Autodesk Inventor part; units mm, degrees
(part 4 of 11)
  arc A1128 (24.4226, 30.9245) -> (24.4226, 30.8483) centre (24.4226, 30.8864) ccw
  arc A1129 (26.162, 30.8483) -> (26.162, 30.9245) centre (26.162, 30.8864) ccw
  line L564 (26.3694, 29.6455) -> (26.2829, 28.3315)
  arc A1130 (26.2448, 28.334) -> (26.3209, 28.329) centre (26.2829, 28.3315) ccw
  arc A1131 (26.3694, 29.6074) -> (26.3694, 29.6836) centre (26.3694, 29.6455) ccw
  line L565 (26.162, 31.0388) -> (24.8504, 31.0388)
  arc A1132 (24.8504, 31.0769) -> (24.8504, 31.0007) centre (24.8504, 31.0388) ccw
  arc A1133 (26.162, 31.0007) -> (26.162, 31.0769) centre (26.162, 31.0388) ccw
  line L566 (26.1708, 28.9489) -> (26.1308, 28.3415)
  arc A1134 (26.0928, 28.344) -> (26.1688, 28.339) centre (26.1308, 28.3415) ccw
  arc A1135 (26.1708, 28.9108) -> (26.1708, 28.987) centre (26.1708, 28.9489) ccw
  line L567 (26.162, 31.1912) -> (25.5924, 31.1912)
  arc A1136 (25.5924, 31.2293) -> (25.5924, 31.1531) centre (25.5924, 31.1912) ccw
  arc A1137 (26.162, 31.1531) -> (26.162, 31.2293) centre (26.162, 31.1912) ccw
  line L568 (5.588, 26.3398) -> (5.6423, 26.9905)
  arc A1138 (5.6803, 26.9873) -> (5.6043, 26.9937) centre (5.6423, 26.9905) ccw
  arc A1139 (5.55, 26.343) -> (5.626, 26.3366) centre (5.588, 26.3398) ccw
  line L569 (5.6423, 26.9905) -> (5.7811, 27.6286)
  arc A1140 (5.8183, 27.6205) -> (5.7439, 27.6366) centre (5.7811, 27.6286) ccw
  arc A1141 (5.6051, 26.9986) -> (5.6795, 26.9824) centre (5.6423, 26.9905) ccw
  line L570 (5.7811, 27.6286) -> (6.0019, 28.243)
  arc A1142 (6.0378, 28.2302) -> (5.9661, 28.2559) centre (6.002, 28.243) ccw
  arc A1143 (5.7452, 27.6414) -> (5.8169, 27.6157) centre (5.7811, 27.6286) ccw
  line L571 (6.0019, 28.243) -> (6.3011, 28.8234)
  arc A1144 (6.335, 28.806) -> (6.2673, 28.8409) centre (6.3011, 28.8234) ccw
  arc A1145 (5.9681, 28.2605) -> (6.0358, 28.2256) centre (6.0019, 28.243) ccw
  line L572 (6.3011, 28.8234) -> (6.6735, 29.3598)
  arc A1146 (6.7048, 29.3381) -> (6.6422, 29.3815) centre (6.6735, 29.3598) ccw
  arc A1147 (6.2698, 28.8452) -> (6.3324, 28.8017) centre (6.3011, 28.8234) ccw
  line L573 (6.6735, 29.3598) -> (7.1127, 29.843)
  arc A1148 (7.1409, 29.8174) -> (7.0845, 29.8686) centre (7.1127, 29.843) ccw
  arc A1149 (6.6453, 29.3854) -> (6.7017, 29.3342) centre (6.6735, 29.3598) ccw
  line L574 (7.1127, 29.843) -> (7.6112, 30.2647)
  arc A1150 (7.6358, 30.2356) -> (7.5866, 30.2938) centre (7.6112, 30.2647) ccw
  arc A1151 (7.0881, 29.8721) -> (7.1373, 29.8139) centre (7.1127, 29.843) ccw
  line L575 (7.6112, 30.2647) -> (8.1605, 30.6178)
  arc A1152 (8.1811, 30.5857) -> (8.1399, 30.6498) centre (8.1605, 30.6178) ccw
  arc A1153 (7.5906, 30.2968) -> (7.6318, 30.2327) centre (7.6112, 30.2647) ccw
  line L576 (8.1605, 30.6178) -> (8.7512, 30.8961)
  arc A1154 (8.7674, 30.8616) -> (8.7349, 30.9305) centre (8.7511, 30.8961) ccw
  arc A1155 (8.1443, 30.6522) -> (8.1768, 30.5833) centre (8.1605, 30.6178) ccw
  line L577 (8.7512, 30.8961) -> (9.3731, 31.0949)
  arc A1156 (9.3847, 31.0586) -> (9.3615, 31.1312) centre (9.3731, 31.0949) ccw
  arc A1157 (8.7395, 30.9324) -> (8.7627, 30.8598) centre (8.7511, 30.8961) ccw
  line L578 (9.3731, 31.0949) -> (10.0157, 31.2112)
  arc A1158 (10.0224, 31.1737) -> (10.0089, 31.2487) centre (10.0157, 31.2112) ccw
  arc A1159 (9.3663, 31.1324) -> (9.3798, 31.0574) centre (9.3731, 31.0949) ccw
  line L579 (10.0157, 31.2112) -> (10.6676, 31.2441)
  arc A1160 (10.6694, 31.206) -> (10.6658, 31.2821) centre (10.6676, 31.2441) ccw
  arc A1161 (10.0138, 31.2493) -> (10.0175, 31.1731) centre (10.0157, 31.2112) ccw
  line L580 (10.6676, 31.2441) -> (11.2768, 31.2186)
  arc A1162 (11.2731, 31.1809) -> (11.2777, 31.257) centre (11.2754, 31.2189) ccw
  arc A1163 (10.6699, 31.2821) -> (10.6653, 31.2061) centre (10.6676, 31.2441) ccw
  line L581 (11.2768, 31.2186) -> (11.8753, 31.0912)
  arc A1164 (11.8769, 31.0569) -> (11.8906, 31.1319) centre (11.8837, 31.0944) ccw
  arc A1165 (11.2822, 31.2564) -> (11.2685, 31.1815) centre (11.2754, 31.2189) ccw
  line L582 (11.8753, 31.0912) -> (12.4777, 30.9778)
  arc A1166 (12.4664, 30.9414) -> (12.489, 31.0142) centre (12.4777, 30.9778) ccw
  arc A1167 (11.8867, 31.1275) -> (11.864, 31.0548) centre (11.8753, 31.0912) ccw
  line L583 (12.4777, 30.9778) -> (12.9624, 30.6072)
  arc A1168 (12.9467, 30.5724) -> (12.978, 30.6419) centre (12.9624, 30.6072) ccw
  arc A1169 (12.4933, 31.0126) -> (12.462, 30.9431) centre (12.4777, 30.9778) ccw
  line L584 (12.9624, 30.6072) -> (14.3509, 26.7983)
  arc A1170 (14.3312, 26.7657) -> (14.3707, 26.8309) centre (14.3509, 26.7983) ccw
  arc A1171 (12.9821, 30.6398) -> (12.9427, 30.5746) centre (12.9624, 30.6072) ccw
  line L585 (14.3509, 26.7983) -> (23.3981, 15.1516)
  arc A1172 (23.4282, 15.1749) -> (23.4216, 15.1816) centre (23.3981, 15.1516) ccw
  arc A1173 (14.3744, 26.8283) -> (14.3274, 26.7683) centre (14.3509, 26.7983) ccw
  line L586 (23.3981, 15.1516) -> (19.5097, 19.7125)
  arc A1174 (16.8769, 22.7269) -> (16.8787, 22.7253) centre (16.8517, 22.6983) ccw
  arc A1175 (23.3654, 15.132) -> (23.3711, 15.1246) centre (23.3981, 15.1516) ccw
  line L587 (19.5097, 19.7125) -> (16.4438, 23.1565)
  arc A1176 (16.4139, 23.1331) -> (16.4738, 23.18) centre (16.4438, 23.1565) ccw
  arc A1177 (16.8233, 22.673) -> (16.8217, 22.6748) centre (16.8517, 22.6983) ccw
  line L588 (16.4438, 23.1565) -> (16.0942, 23.6606)
  arc A1178 (16.0616, 23.6409) -> (16.1268, 23.6803) centre (16.0942, 23.6606) ccw
  arc A1179 (16.4765, 23.1763) -> (16.4112, 23.1368) centre (16.4438, 23.1565) ccw
  line L589 (16.0942, 23.6606) -> (15.8078, 24.2031)
  arc A1180 (15.7731, 24.1874) -> (15.8426, 24.2187) centre (15.8078, 24.2031) ccw
  arc A1181 (16.1289, 23.6762) -> (16.0594, 23.6449) centre (16.0942, 23.6606) ccw
  line L590 (15.8078, 24.2031) -> (15.5889, 24.7761)
  arc A1182 (15.5525, 24.7648) -> (15.6253, 24.7875) centre (15.5889, 24.7761) ccw
  arc A1183 (15.8442, 24.2144) -> (15.7714, 24.1917) centre (15.8078, 24.2031) ccw
  line L591 (15.5889, 24.7761) -> (15.4407, 25.3714)
  arc A1184 (15.4032, 25.3645) -> (15.4781, 25.3783) centre (15.4407, 25.3714) ccw
  arc A1185 (15.6379, 27.3846) -> (15.5629, 27.3709) centre (15.6004, 27.3777) ccw
  line L592 (15.4407, 25.3714) -> (14.9039, 25.4351)
  arc A1186 (14.8659, 25.4328) -> (14.942, 25.4374) centre (14.9039, 25.4351) ccw
  arc A1187 (15.4787, 25.3737) -> (15.4026, 25.3691) centre (15.4407, 25.3714) ccw
  line L593 (14.9039, 25.4351) -> (18.8583, 22.6449)
  arc A1188 (18.8203, 22.6472) -> (18.8963, 22.6426) centre (18.8583, 22.6449) ccw
  arc A1189 (14.942, 25.4328) -> (14.8659, 25.4374) centre (14.9039, 25.4351) ccw
  line L594 (18.8583, 22.6449) -> (13.5985, 27.0666)
  arc A1190 (15.5629, 24.9531) -> (15.6379, 24.9394) centre (15.6004, 24.9463) ccw
  arc A1191 (18.8958, 22.638) -> (18.8208, 22.6517) centre (18.8583, 22.6449) ccw
  line L595 (13.5985, 27.0666) -> (5.328, 28.9324)
  arc A1192 (5.2916, 28.9437) -> (5.3643, 28.9211) centre (5.328, 28.9324) ccw
  arc A1193 (13.6349, 27.0553) -> (13.5621, 27.0779) centre (13.5985, 27.0666) ccw
  line L596 (5.328, 28.9324) -> (19.749, 27.0115)
  arc A1194 (5.9013, 28.867) -> (5.9708, 28.8358) centre (5.936, 28.8514) ccw
  arc A1195 (5.3627, 28.9167) -> (5.2932, 28.948) centre (5.328, 28.9324) ccw
  line L597 (19.749, 27.0115) -> (10.434, 29.4468)
  arc A1196 (10.4014, 29.4665) -> (10.4666, 29.4271) centre (10.434, 29.4468) ccw
  arc A1197 (19.7816, 26.9918) -> (19.7164, 27.0312) centre (19.749, 27.0115) ccw
  line L598 (10.434, 29.4468) -> (20.7175, 25.3208)
  arc A1198 (10.9892, 29.183) -> (11.0176, 29.2538) centre (11.0034, 29.2184) ccw
  arc A1199 (10.464, 29.4233) -> (10.404, 29.4703) centre (10.434, 29.4468) ccw
  line L599 (20.7175, 25.3208) -> (12.0354, 22.6782)
  arc A1200 (12.0377, 22.6402) -> (12.0332, 22.7163) centre (12.0354, 22.6782) ccw
  arc A1201 (11.0303, 29.1914) -> (10.9764, 29.2453) centre (11.0034, 29.2184) ccw
  line L600 (12.0354, 22.6782) -> (14.4431, 22.5281)
  arc A1202 (14.4196, 22.5581) -> (14.4666, 22.4982) centre (14.4431, 22.5281) ccw
  arc A1203 (12.0589, 22.6482) -> (12.0119, 22.7082) centre (12.0354, 22.6782) ccw
  line L601 (14.4431, 22.5281) -> (13.0207, 21.6798)
  arc A1204 (13.001, 21.7124) -> (13.0404, 21.6472) centre (13.0207, 21.6798) ccw
  arc A1205 (14.4628, 22.4955) -> (14.4234, 22.5608) centre (14.4431, 22.5281) ccw
  line L602 (13.0207, 21.6798) -> (12.4691, 21.4111)
  arc A1206 (12.4535, 21.4459) -> (12.4848, 21.3764) centre (12.4691, 21.4111) ccw
  arc A1207 (13.0363, 21.645) -> (13.005, 21.7145) centre (13.0207, 21.6798) ccw
  line L603 (12.4691, 21.4111) -> (11.8832, 21.2297)
  arc A1208 (11.8719, 21.2661) -> (11.8946, 21.1933) centre (11.8832, 21.2297) ccw
  arc A1209 (12.4805, 21.3748) -> (12.4578, 21.4475) centre (12.4691, 21.4111) ccw
  line L604 (11.8832, 21.2297) -> (11.28, 21.1185)
  arc A1210 (11.2731, 21.156) -> (11.2868, 21.081) centre (11.28, 21.1185) ccw
  arc A1211 (11.8906, 21.1921) -> (11.8769, 21.2671) centre (11.8837, 21.2296) ccw
  line L605 (11.28, 21.1185) -> (10.668, 21.0819)
  arc A1212 (10.6657, 21.1199) -> (10.6703, 21.0439) centre (10.668, 21.0819) ccw
  arc A1213 (11.2823, 21.0805) -> (11.2777, 21.1565) centre (11.28, 21.1185) ccw
  line L606 (10.668, 21.0819) -> (10.0106, 21.1406)
  arc A1214 (10.014, 21.1786) -> (10.0072, 21.1027) centre (10.0106, 21.1406) ccw
  arc A1215 (10.6646, 21.044) -> (10.6714, 21.1199) centre (10.668, 21.0819) ccw
  line L607 (10.0106, 21.1406) -> (9.3659, 21.2818)
  arc A1216 (9.3741, 21.319) -> (9.3578, 21.2446) centre (9.3659, 21.2818) ccw
  arc A1217 (10.0025, 21.1034) -> (10.0188, 21.1778) centre (10.0106, 21.1406) ccw
  line L608 (9.3659, 21.2818) -> (8.7436, 21.502)
  arc A1218 (8.7565, 21.5379) -> (8.7308, 21.4661) centre (8.7436, 21.502) ccw
  arc A1219 (9.3532, 21.2459) -> (9.3787, 21.3177) centre (9.3659, 21.2818) ccw
  line L609 (8.7436, 21.502) -> (8.1556, 21.8016)
  arc A1220 (8.1727, 21.8355) -> (8.1383, 21.7675) centre (8.1555, 21.8015) ccw
  arc A1221 (8.7264, 21.468) -> (8.7608, 21.536) centre (8.7436, 21.502) ccw
  line L610 (8.1556, 21.8016) -> (7.6091, 22.1716)
  arc A1222 (7.6305, 22.2032) -> (7.5877, 22.1401) centre (7.6091, 22.1716) ccw
  arc A1223 (8.1341, 21.7699) -> (8.1768, 21.833) centre (8.1555, 21.8015) ccw
  line L611 (7.6091, 22.1716) -> (7.1138, 22.6078)
  arc A1224 (7.139, 22.6364) -> (7.0887, 22.5793) centre (7.1138, 22.6078) ccw
  arc A1225 (7.5839, 22.143) -> (7.6343, 22.2002) centre (7.6091, 22.1716) ccw
  line L612 (7.1138, 22.6078) -> (6.6776, 23.1031)
  arc A1226 (6.7062, 23.1283) -> (6.649, 23.0779) centre (6.6776, 23.1031) ccw
  arc A1227 (7.0853, 22.5827) -> (7.1424, 22.633) centre (7.1138, 22.6078) ccw
  line L613 (6.6776, 23.1031) -> (6.3075, 23.6495)
  arc A1228 (6.339, 23.6708) -> (6.2759, 23.6281) centre (6.3075, 23.6495) ccw
  arc A1229 (6.6461, 23.0817) -> (6.7092, 23.1245) centre (6.6776, 23.1031) ccw
  line L614 (6.3075, 23.6495) -> (6.0093, 24.2382)
  arc A1230 (6.0432, 24.2554) -> (5.9753, 24.221) centre (6.0093, 24.2382) ccw
  arc A1231 (6.2735, 23.6323) -> (6.3415, 23.6667) centre (6.3075, 23.6495) ccw
  line L615 (6.0093, 24.2382) -> (5.7878, 24.8599)
  arc A1232 (5.8237, 24.8727) -> (5.7519, 24.8472) centre (5.7878, 24.8599) ccw
  arc A1233 (5.9734, 24.2254) -> (6.0451, 24.251) centre (6.0093, 24.2382) ccw
  line L616 (5.7878, 24.8599) -> (5.6466, 25.5046)
  arc A1234 (5.6838, 25.5128) -> (5.6094, 25.4965) centre (5.6466, 25.5046) ccw
  arc A1235 (5.7506, 24.8518) -> (5.825, 24.8681) centre (5.7878, 24.8599) ccw
  line L617 (5.6466, 25.5046) -> (5.588, 26.162)
  arc A1236 (5.6259, 26.1654) -> (5.5501, 26.1586) centre (5.588, 26.162) ccw
  arc A1237 (5.6087, 25.5012) -> (5.6846, 25.508) centre (5.6466, 25.5046) ccw
  line L618 (5.588, 26.162) -> (6.858, 26.162)
  arc A1238 (6.858, 26.1239) -> (6.858, 26.2001) centre (6.858, 26.162) ccw
  arc A1239 (5.588, 26.2001) -> (5.588, 26.1239) centre (5.588, 26.162) ccw
  line L619 (6.858, 26.162) -> (6.8774, 25.6365)
  arc A1240 (6.8393, 25.6351) -> (6.9155, 25.638) centre (6.8774, 25.6366) ccw
  arc A1241 (6.8961, 26.1634) -> (6.8199, 26.1606) centre (6.858, 26.162) ccw
  line L620 (6.8774, 25.6365) -> (6.9714, 25.1192)
  arc A1242 (6.9339, 25.1124) -> (7.0089, 25.126) centre (6.9714, 25.1192) ccw
  arc A1243 (6.9149, 25.6434) -> (6.8399, 25.6297) centre (6.8774, 25.6366) ccw
  line L621 (6.9714, 25.1192) -> (7.1381, 24.6205)
  arc A1244 (7.1019, 24.6085) -> (7.1742, 24.6326) centre (7.1381, 24.6206) ccw
  arc A1245 (7.0075, 25.1313) -> (6.9353, 25.1072) centre (6.9714, 25.1192) ccw
  line L622 (7.1381, 24.6205) -> (7.374, 24.1506)
  arc A1246 (7.34, 24.1335) -> (7.4081, 24.1677) centre (7.374, 24.1506) ccw
  arc A1247 (7.1721, 24.6376) -> (7.104, 24.6035) centre (7.1381, 24.6206) ccw
  line L623 (7.374, 24.1506) -> (7.6744, 23.7191)
  arc A1248 (7.6431, 23.6973) -> (7.7057, 23.7409) centre (7.6744, 23.7191) ccw
  arc A1249 (7.4053, 24.1724) -> (7.3427, 24.1289) centre (7.374, 24.1506) ccw
  line L624 (7.6744, 23.7191) -> (8.0332, 23.3347)
  arc A1250 (8.0053, 23.3087) -> (8.061, 23.3607) centre (8.0332, 23.3347) ccw
  arc A1251 (7.7023, 23.7451) -> (7.6465, 23.6931) centre (7.6744, 23.7191) ccw
  line L625 (8.0332, 23.3347) -> (8.443, 23.0053)
  arc A1252 (8.4191, 22.9756) -> (8.4669, 23.035) centre (8.443, 23.0053) ccw
  arc A1253 (8.057, 23.3644) -> (8.0093, 23.305) centre (8.0332, 23.3347) ccw
  line L626 (8.443, 23.0053) -> (8.8955, 22.7376)
  arc A1254 (8.8761, 22.7048) -> (8.9149, 22.7704) centre (8.8955, 22.7376) ccw
  arc A1255 (8.4624, 23.0381) -> (8.4236, 22.9725) centre (8.443, 23.0053) ccw
  line L627 (8.8955, 22.7376) -> (9.3815, 22.537)
  arc A1256 (9.367, 22.5018) -> (9.3961, 22.5722) centre (9.3815, 22.537) ccw
  arc A1257 (8.91, 22.7728) -> (8.881, 22.7024) centre (8.8955, 22.7376) ccw
  line L628 (9.3815, 22.537) -> (9.8911, 22.4076)
  arc A1258 (9.8818, 22.3706) -> (9.9005, 22.4445) centre (9.8911, 22.4076) ccw
  arc A1259 (9.3909, 22.5739) -> (9.3721, 22.5) centre (9.3815, 22.537) ccw
  line L629 (9.8911, 22.4076) -> (10.414, 22.352)
  arc A1260 (10.41, 22.3141) -> (10.418, 22.3899) centre (10.414, 22.352) ccw
  arc A1261 (9.8952, 22.4455) -> (9.8871, 22.3697) centre (9.8911, 22.4076) ccw
  line L630 (10.414, 22.352) -> (10.6681, 22.3519)
  arc A1262 (10.6681, 22.3138) -> (10.6681, 22.39) centre (10.6681, 22.3519) ccw
  arc A1263 (10.414, 22.3901) -> (10.414, 22.3139) centre (10.414, 22.352) ccw
  line L631 (10.6681, 22.3519) -> (11.2103, 22.3905)
  arc A1264 (11.213, 22.3525) -> (11.2076, 22.4285) centre (11.2103, 22.3905) ccw
  arc A1265 (10.6653, 22.3899) -> (10.6708, 22.3139) centre (10.6681, 22.3519) ccw
  line L632 (11.2103, 22.3905) -> (11.7415, 22.5058)
  arc A1266 (11.7496, 22.4686) -> (11.7334, 22.543) centre (11.7415, 22.5058) ccw
  arc A1267 (11.2022, 22.4277) -> (11.2184, 22.3532) centre (11.2103, 22.3905) ccw
  line L633 (11.7415, 22.5058) -> (12.2509, 22.6955)
  arc A1268 (12.264, 22.6606) -> (12.2374, 22.732) centre (12.2507, 22.6963) ccw
  arc A1269 (11.7282, 22.5415) -> (11.7548, 22.4701) centre (11.7415, 22.5058) ccw
  line L634 (12.2509, 22.6955) -> (12.7282, 22.9558)
  arc A1270 (12.7464, 22.9224) -> (12.7099, 22.9893) centre (12.7282, 22.9558) ccw
  arc A1271 (12.2325, 22.7297) -> (12.269, 22.6629) centre (12.2507, 22.6963) ccw
  line L635 (12.7282, 22.9558) -> (12.9175, 23.4562)
  arc A1272 (13.1859, 23.2521) -> (13.1402, 23.3131) centre (13.163, 23.2826) ccw
  arc A1273 (12.7053, 22.9863) -> (12.751, 22.9253) centre (12.7282, 22.9558) ccw
  line L636 (12.9175, 23.4562) -> (13.0355, 23.9868)
  arc A1274 (13.5743, 23.64) -> (13.5205, 23.6939) centre (13.5474, 23.667) ccw
  arc A1275 (13.1361, 23.3095) -> (13.19, 23.2557) centre (13.163, 23.2826) ccw
  line L637 (13.0355, 23.9868) -> (13.0769, 24.5288)
  arc A1276 (13.1074, 24.506) -> (13.0464, 24.5517) centre (13.0769, 24.5288) ccw
  arc A1277 (13.5169, 23.6898) -> (13.5779, 23.6441) centre (13.5474, 23.667) ccw
  line L638 (13.0769, 24.5288) -> (13.0407, 25.0712)
  arc A1278 (14.1671, 24.561) -> (14.1003, 24.5975) centre (14.1337, 24.5793) ccw
  arc A1279 (13.0435, 24.5471) -> (13.1103, 24.5106) centre (13.0769, 24.5288) ccw
  line L639 (13.0407, 25.0712) -> (12.9277, 25.6029)
  arc A1280 (12.9633, 25.5896) -> (12.892, 25.6162) centre (12.9277, 25.6029) ccw
  arc A1281 (14.098, 24.5926) -> (14.1694, 24.566) centre (14.1337, 24.5793) ccw
  line L640 (12.9277, 25.6029) -> (22.6056, 27.554)
  arc A1282 (22.6429, 27.5459) -> (22.5684, 27.5621) centre (22.6056, 27.554) ccw
  arc A1283 (12.8904, 25.611) -> (12.9649, 25.5948) centre (12.9277, 25.6029) ccw
  line L641 (22.6056, 27.554) -> (9.5434, 30.1539)
  arc A1284 (9.5814, 30.1512) -> (9.5054, 30.1566) centre (9.5434, 30.1539) ccw
  arc A1285 (22.5676, 27.5568) -> (22.6436, 27.5513) centre (22.6056, 27.554) ccw
  line L642 (9.5434, 30.1539) -> (9.9852, 30.1292)
  arc A1286 (10.0232, 30.1319) -> (9.9472, 30.1265) centre (9.9852, 30.1292) ccw
  arc A1287 (9.5054, 30.1512) -> (9.5814, 30.1566) centre (9.5434, 30.1539) ccw
  line L643 (9.9852, 30.1292) -> (10.4403, 29.8319)
  arc A1288 (10.4775, 29.84) -> (10.403, 29.8238) centre (10.4403, 29.8319) ccw
  arc A1289 (9.9479, 30.1211) -> (10.0224, 30.1373) centre (9.9852, 30.1292) ccw
  line L644 (10.4403, 29.8319) -> (10.9331, 29.6024)
  arc A1290 (14.1694, 27.758) -> (14.098, 27.7314) centre (14.1337, 27.7447) ccw
  arc A1291 (10.4046, 29.8186) -> (10.476, 29.8452) centre (10.4403, 29.8319) ccw
  line L645 (10.9331, 29.6024) -> (11.4535, 29.4454)
  arc A1292 (11.4869, 29.4637) -> (11.42, 29.4271) centre (11.4535, 29.4454) ccw
  arc A1293 (14.1003, 27.7265) -> (14.1671, 27.763) centre (14.1337, 27.7447) ccw
  line L646 (11.4535, 29.4454) -> (11.991, 29.364)
  arc A1294 (13.5779, 28.6799) -> (13.5169, 28.6342) centre (13.5474, 28.657) ccw
  arc A1295 (11.423, 29.4226) -> (11.484, 29.4682) centre (11.4535, 29.4454) ccw
  line L647 (11.991, 29.364) -> (12.5346, 29.36)
  arc A1296 (13.19, 29.0683) -> (13.1361, 29.0145) centre (13.163, 29.0414) ccw
  arc A1297 (13.5205, 28.6301) -> (13.5743, 28.684) centre (13.5474, 28.657) ccw
  line L648 (12.5346, 29.36) -> (12.7342, 29.3872)
  arc A1298 (12.7571, 29.4177) -> (12.7114, 29.3567) centre (12.7342, 29.3872) ccw
  arc A1299 (13.1402, 29.0109) -> (13.1859, 29.0719) centre (13.163, 29.0414) ccw
  line L649 (12.7342, 29.3872) -> (12.2551, 29.6441)
  arc A1300 (12.269, 29.6611) -> (12.2325, 29.5943) centre (12.2507, 29.6277) ccw
  arc A1301 (12.716, 29.3537) -> (12.7525, 29.4206) centre (12.7342, 29.3872) ccw
  line L650 (12.2551, 29.6441) -> (11.7444, 29.8301)
  arc A1302 (11.7577, 29.8658) -> (11.7311, 29.7945) centre (11.7444, 29.8301) ccw
  arc A1303 (12.2374, 29.592) -> (12.264, 29.6634) centre (12.2507, 29.6277) ccw
  line L651 (11.7444, 29.8301) -> (11.2123, 29.9416)
  arc A1304 (11.2204, 29.9789) -> (11.2042, 29.9044) centre (11.2123, 29.9416) ccw
  arc A1305 (11.7363, 29.7929) -> (11.7525, 29.8674) centre (11.7444, 29.8301) ccw
  line L652 (11.2123, 29.9416) -> (10.6698, 29.9763)
  arc A1306 (10.6726, 30.0143) -> (10.6671, 29.9383) centre (10.6698, 29.9763) ccw
  arc A1307 (11.2096, 29.9036) -> (11.2151, 29.9796) centre (11.2123, 29.9416) ccw
  line L653 (10.6698, 29.9763) -> (10.1821, 29.9523)
  arc A1308 (10.18, 29.9898) -> (10.1831, 29.9137) centre (10.1815, 29.9518) ccw
  arc A1309 (10.6714, 29.9382) -> (10.6683, 30.0144) centre (10.6698, 29.9763) ccw
  line L654 (10.1821, 29.9523) -> (9.7019, 29.8682)
  arc A1310 (9.6953, 29.9058) -> (9.7084, 29.8307) centre (9.7019, 29.8682) ccw
  arc A1311 (10.1881, 29.9142) -> (10.175, 29.9893) centre (10.1815, 29.9518) ccw
  line L655 (9.7019, 29.8682) -> (9.2372, 29.7228)
  arc A1312 (9.2258, 29.7591) -> (9.2486, 29.6864) centre (9.2372, 29.7228) ccw
  arc A1313 (9.7133, 29.8318) -> (9.6905, 29.9046) centre (9.7019, 29.8682) ccw
  line L656 (9.2372, 29.7228) -> (8.7955, 29.518)
  arc A1314 (8.7795, 29.5525) -> (8.8116, 29.4834) centre (8.7955, 29.5179) ccw
  arc A1315 (9.2533, 29.6882) -> (9.2212, 29.7573) centre (9.2372, 29.7228) ccw
  line L657 (8.7955, 29.518) -> (8.3843, 29.2572)
  arc A1316 (8.3639, 29.2894) -> (8.4047, 29.225) centre (8.3843, 29.2572) ccw
  arc A1317 (8.8159, 29.4857) -> (8.7751, 29.5501) centre (8.7955, 29.5179) ccw
  line L658 (8.3843, 29.2572) -> (8.0107, 28.945)
  arc A1318 (7.9863, 28.9742) -> (8.0352, 28.9157) centre (8.0107, 28.945) ccw
  arc A1319 (8.4088, 29.228) -> (8.3599, 29.2864) centre (8.3843, 29.2572) ccw
  line L659 (8.0107, 28.945) -> (7.6811, 28.5867)
  arc A1320 (7.653, 28.6125) -> (7.7091, 28.5609) centre (7.6811, 28.5867) ccw
  arc A1321 (8.0388, 28.9192) -> (7.9827, 28.9708) centre (8.0107, 28.945) ccw
  line L660 (7.6811, 28.5867) -> (7.401, 28.1884)
  arc A1322 (7.3698, 28.2104) -> (7.4321, 28.1665) centre (7.401, 28.1884) ccw
  arc A1323 (7.7122, 28.5648) -> (7.6499, 28.6086) centre (7.6811, 28.5867) ccw
  line L661 (7.401, 28.1884) -> (7.1753, 27.757)
  arc A1324 (7.1415, 27.7747) -> (7.209, 27.7394) centre (7.1753, 27.757) ccw
  arc A1325 (7.4347, 28.1708) -> (7.3672, 28.2061) centre (7.401, 28.1884) ccw
  line L662 (7.1753, 27.757) -> (7.6204, 27.5599)
  arc A1326 (6.972, 27.313) -> (7.0436, 27.2868) centre (7.0078, 27.2999) ccw
  arc A1327 (7.211, 27.7439) -> (7.1395, 27.7702) centre (7.1753, 27.757) ccw
  line L663 (7.6204, 27.5599) -> (6.9014, 26.8247)
  arc A1328 (6.8642, 26.8331) -> (6.9386, 26.8164) centre (6.9014, 26.8247) ccw
  arc A1329 (12.9568, 32.9698) -> (12.8825, 32.9865) centre (12.9197, 32.9781) ccw
  line L664 (6.9014, 26.8247) -> (6.858, 26.3398)
  arc A1330 (6.8201, 26.3432) -> (6.8959, 26.3364) centre (6.858, 26.3398) ccw
  arc A1331 (6.9394, 26.8213) -> (6.8635, 26.8281) centre (6.9014, 26.8247) ccw
  line L665 (6.858, 26.3398) -> (5.588, 26.3398)
  arc A1332 (5.588, 26.3779) -> (5.588, 26.3017) centre (5.588, 26.3398) ccw
  arc A1333 (6.858, 26.3017) -> (6.858, 26.3779) centre (6.858, 26.3398) ccw
  line L666 (15.4591, 25.2973) -> (14.7422, 26.1051)
  arc A1334 (14.7041, 26.1051) -> (14.7803, 26.1051) centre (14.7422, 26.1051) ccw
  arc A1335 (15.4972, 25.2973) -> (15.421, 25.2973) centre (15.4591, 25.2973) ccw
  line L667 (15.6556, 24.6016) -> (14.6713, 26.8246)
  arc A1336 (14.6332, 26.8246) -> (14.7094, 26.8246) centre (14.6713, 26.8246) ccw
  arc A1337 (15.6937, 24.6016) -> (15.6175, 24.6016) centre (15.6556, 24.6016) ccw
  line L668 (15.8368, 24.1482) -> (5.3895, 28.9242)
  arc A1338 (5.3514, 28.9242) -> (5.4276, 28.9242) centre (5.3895, 28.9242) ccw
  arc A1339 (15.8749, 24.1482) -> (15.7987, 24.1482) centre (15.8368, 24.1482) ccw
  line L669 (16.0101, 23.8198) -> (14.7162, 27.6819)
  arc A1340 (14.6781, 27.6819) -> (14.7543, 27.6819) centre (14.7162, 27.6819) ccw
  arc A1341 (16.0482, 23.8198) -> (15.972, 23.8198) centre (16.0101, 23.8198) ccw
  line L670 (16.1807, 23.5359) -> (19.6022, 27.0499)
  arc A1342 (19.5641, 27.0499) -> (19.6403, 27.0499) centre (19.6022, 27.0499) ccw
  arc A1343 (16.2188, 23.5359) -> (16.1426, 23.5359) centre (16.1807, 23.5359) ccw
  line L671 (16.3486, 23.2938) -> (14.8395, 28.295)
  arc A1344 (14.8014, 28.295) -> (14.8776, 28.295) centre (14.8395, 28.295) ccw
  arc A1345 (16.3867, 23.2938) -> (16.3105, 23.2938) centre (16.3486, 23.2938) ccw
  line L672 (16.515, 23.0767) -> (16.1422, 29.0049)
  arc A1346 (16.1041, 29.0049) -> (16.1803, 29.0049) centre (16.1422, 29.0049) ccw
  arc A1347 (16.5531, 23.0767) -> (16.4769, 23.0767) centre (16.515, 23.0767) ccw
  line L673 (16.6793, 22.8921) -> (10.7626, 29.315)
  arc A1348 (10.7245, 29.315) -> (10.8007, 29.315) centre (10.7626, 29.315) ccw
  arc A1349 (16.7174, 22.8921) -> (16.6412, 22.8921) centre (16.6793, 22.8921) ccw
  line L674 (12.0171, 28.1294) -> (9.5434, 30.1539)
  arc A1350 (9.5053, 30.1539) -> (9.5815, 30.1539) centre (9.5434, 30.1539) ccw
  arc A1351 (12.0552, 28.1294) -> (11.979, 28.1294) centre (12.0171, 28.1294) ccw
  line L675 (9.5434, 30.1539) -> (9.9028, 29.66)
  arc A1352 (9.8647, 29.66) -> (9.9409, 29.66) centre (9.9028, 29.66) ccw
  arc A1353 (9.5815, 30.1539) -> (9.5053, 30.1539) centre (9.5434, 30.1539) ccw
  line L676 (19.6426, 19.5567) -> (10.4327, 29.8369)
  arc A1354 (10.3946, 29.8369) -> (10.4708, 29.8369) centre (10.4327, 29.8369) ccw
  arc A1355 (19.6807, 19.5567) -> (19.6045, 19.5567) centre (19.6426, 19.5567) ccw
  line L677 (21.7522, 27.382) -> (20.5215, 25.2612)
  arc A1356 (20.4834, 25.2612) -> (20.5596, 25.2612) centre (20.5215, 25.2612) ccw
  arc A1357 (21.7903, 27.382) -> (21.7141, 27.382) centre (21.7522, 27.382) ccw
  line L678 (12.3669, 28.0907) -> (10.8306, 29.6501)
  arc A1358 (10.7925, 29.6501) -> (10.8687, 29.6501) centre (10.8306, 29.6501) ccw
  arc A1359 (12.405, 28.0907) -> (12.3288, 28.0907) centre (12.3669, 28.0907) ccw
  line L679 (13.0172, 25.1818) -> (14.192, 23.3346)
  arc A1360 (14.1539, 23.3346) -> (14.2301, 23.3346) centre (14.192, 23.3346) ccw
  arc A1361 (13.0553, 25.1818) -> (12.9791, 25.1818) centre (13.0172, 25.1818) ccw
  line L680 (12.58, 28.0916) -> (11.1586, 29.5344)
  arc A1362 (11.1205, 29.5344) -> (11.1967, 29.5344) centre (11.1586, 29.5344) ccw
  arc A1363 (12.6181, 28.0916) -> (12.5419, 28.0916) centre (12.58, 28.0916) ccw
  line L681 (13.0564, 24.8362) -> (14.1433, 23.1272)
  arc A1364 (14.1052, 23.1272) -> (14.1814, 23.1272) centre (14.1433, 23.1272) ccw
  arc A1365 (13.0945, 24.8362) -> (13.0183, 24.8362) centre (13.0564, 24.8362) ccw
  line L682 (23.5292, 14.9828) -> (11.4614, 29.4442)
  arc A1366 (11.4233, 29.4442) -> (11.4995, 29.4442) centre (11.4614, 29.4442) ccw
  arc A1367 (23.5673, 14.9828) -> (23.4911, 14.9828) centre (23.5292, 14.9828) ccw
  line L683 (13.0763, 24.5209) -> (12.2488, 22.6649)
  arc A1368 (12.2107, 22.6649) -> (12.2869, 22.6649) centre (12.2488, 22.6649) ccw
  arc A1369 (13.1144, 24.5209) -> (13.0382, 24.5209) centre (13.0763, 24.5209) ccw
  line L684 (23.648, 14.8299) -> (11.7128, 29.4061)
  arc A1370 (11.6747, 29.4061) -> (11.7509, 29.4061) centre (11.7128, 29.4061) ccw
  arc A1371 (23.6861, 14.8299) -> (23.6099, 14.8299) centre (23.648, 14.8299) ccw
  line L685 (13.0569, 24.2673) -> (12.442, 22.6529)
  arc A1372 (12.4039, 22.6529) -> (12.4801, 22.6529) centre (12.442, 22.6529) ccw
  arc A1373 (13.095, 24.2673) -> (13.0188, 24.2673) centre (13.0569, 24.2673) ccw
  line L686 (13.278, 28.1796) -> (11.9643, 29.3681)
  arc A1374 (11.9262, 29.3681) -> (12.0024, 29.3681) centre (11.9643, 29.3681) ccw
  arc A1375 (13.3161, 28.1796) -> (13.2399, 28.1796) centre (13.278, 28.1796) ccw
  line L687 (13.0376, 24.0137) -> (13.9419, 22.5594)
  arc A1376 (13.9038, 22.5594) -> (13.98, 22.5594) centre (13.9419, 22.5594) ccw
  arc A1377 (13.0757, 24.0137) -> (12.9995, 24.0137) centre (13.0376, 24.0137) ccw
  line L688 (14.2939, 26.9548) -> (13.2686, 25.6803)
  arc A1378 (13.2305, 25.6803) -> (13.3067, 25.6803) centre (13.2686, 25.6803) ccw
  arc A1379 (14.332, 26.9548) -> (14.2558, 26.9548) centre (14.2939, 26.9548) ccw
  line L689 (14.3098, 24.0785) -> (14.3, 22.4428)
  arc A1380 (14.2619, 22.4428) -> (14.3381, 22.4428) centre (14.3, 22.4428) ccw
  arc A1381 (14.3479, 24.0785) -> (14.2717, 24.0785) centre (14.3098, 24.0785) ccw
  line L690 (14.2329, 27.1221) -> (13.2454, 25.8946)
  arc A1382 (13.2073, 25.8946) -> (13.2835, 25.8946) centre (13.2454, 25.8946) ccw
  arc A1383 (14.271, 27.1221) -> (14.1948, 27.1221) centre (14.2329, 27.1221) ccw
  line L691 (14.1565, 23.927) -> (14.1471, 22.3516)
  arc A1384 (14.109, 22.3516) -> (14.1852, 22.3516) centre (14.1471, 22.3516) ccw
  arc A1385 (14.1946, 23.927) -> (14.1184, 23.927) centre (14.1565, 23.927) ccw
  line L692 (13.7852, 28.3501) -> (12.6046, 29.3695)
  arc A1386 (12.5665, 29.3695) -> (12.6427, 29.3695) centre (12.6046, 29.3695) ccw
  arc A1387 (13.8233, 28.3501) -> (13.7471, 28.3501) centre (13.7852, 28.3501) ccw
  line L693 (12.8925, 23.39) -> (13.6973, 22.0834)
  arc A1388 (13.6592, 22.0834) -> (13.7354, 22.0834) centre (13.6973, 22.0834) ccw
  arc A1389 (12.9306, 23.39) -> (12.8544, 23.39) centre (12.8925, 23.39) ccw
  line L694 (12.8972, 30.657) -> (12.5563, 29.2005)
  arc A1390 (12.5182, 29.2005) -> (12.5944, 29.2005) centre (12.5563, 29.2005) ccw
  arc A1391 (12.9353, 30.657) -> (12.8591, 30.657) centre (12.8972, 30.657) ccw
  line L695 (12.9015, 23.1391) -> (12.9469, 21.6439)
  arc A1392 (12.9088, 21.6439) -> (12.985, 21.6439) centre (12.9469, 21.6439) ccw
  arc A1393 (12.9396, 23.1391) -> (12.8634, 23.1391) centre (12.9015, 23.1391) ccw
  line L696 (12.7645, 30.7585) -> (12.4339, 29.3463)
  arc A1394 (12.3958, 29.3463) -> (12.472, 29.3463) centre (12.4339, 29.3463) ccw
  arc A1395 (12.8026, 30.7585) -> (12.7264, 30.7585) centre (12.7645, 30.7585) ccw
  line L697 (12.7526, 23.0204) -> (12.7967, 21.5707)
  arc A1396 (12.7586, 21.5707) -> (12.8348, 21.5707) centre (12.7967, 21.5707) ccw
  arc A1397 (12.7907, 23.0204) -> (12.7145, 23.0204) centre (12.7526, 23.0204) ccw
  line L698 (12.6444, 30.8503) -> (12.6553, 29.4295)
  arc A1398 (12.6172, 29.4295) -> (12.6934, 29.4295) centre (12.6553, 29.4295) ccw
  arc A1399 (12.6825, 30.8503) -> (12.6063, 30.8503) centre (12.6444, 30.8503) ccw
  line L699 (12.6495, 22.9129) -> (12.6464, 21.4975)
  arc A1400 (12.6083, 21.4975) -> (12.6845, 21.4975) centre (12.6464, 21.4975) ccw
  arc A1401 (12.6876, 22.9129) -> (12.6114, 22.9129) centre (12.6495, 22.9129) ccw
  line L700 (12.4915, 30.9178) -> (12.5022, 29.5116)
  arc A1402 (12.4641, 29.5116) -> (12.5403, 29.5116) centre (12.5022, 29.5116) ccw
  arc A1403 (12.5296, 30.9178) -> (12.4534, 30.9178) centre (12.4915, 30.9178) ccw
  line L701 (12.4971, 22.8298) -> (12.4962, 21.4243)
  arc A1404 (12.4581, 21.4243) -> (12.5343, 21.4243) centre (12.4962, 21.4243) ccw
  arc A1405 (12.5352, 22.8298) -> (12.459, 22.8298) centre (12.4971, 22.8298) ccw
  line L702 (12.3387, 30.9679) -> (12.3492, 29.5936)
  arc A1406 (12.3111, 29.5936) -> (12.3873, 29.5936) centre (12.3492, 29.5936) ccw
  arc A1407 (12.3768, 30.9679) -> (12.3006, 30.9679) centre (12.3387, 30.9679) ccw
  line L703 (12.3446, 22.7466) -> (12.344, 21.3723)
  arc A1408 (12.3059, 21.3723) -> (12.3821, 21.3723) centre (12.344, 21.3723) ccw
  arc A1409 (12.3827, 22.7466) -> (12.3065, 22.7466) centre (12.3446, 22.7466) ccw
  line L704 (12.1921, 31.0316) -> (12.1963, 29.6655)
  arc A1410 (12.1582, 29.6655) -> (12.2344, 29.6655) centre (12.1963, 29.6655) ccw
  arc A1411 (12.2302, 31.0316) -> (12.154, 31.0316) centre (12.1921, 31.0316) ccw
  line L705 (12.1922, 22.6736) -> (12.1916, 21.3252)
  arc A1412 (12.1535, 21.3252) -> (12.2297, 21.3252) centre (12.1916, 21.3252) ccw
  arc A1413 (12.2303, 22.6736) -> (12.1541, 22.6736) centre (12.1922, 22.6736) ccw
  line L706 (12.0334, 31.0614) -> (12.0434, 29.7212)
  arc A1414 (12.0053, 29.7212) -> (12.0815, 29.7212) centre (12.0434, 29.7212) ccw
  arc A1415 (12.0715, 31.0614) -> (11.9953, 31.0614) centre (12.0334, 31.0614) ccw
  line L707 (12.0398, 22.6169) -> (12.039, 21.2779)
  arc A1416 (12.0009, 21.2779) -> (12.0771, 21.2779) centre (12.039, 21.2779) ccw
  arc A1417 (12.0779, 22.6169) -> (12.0017, 22.6169) centre (12.0398, 22.6169) ccw
  line L708 (11.8805, 31.1069) -> (11.8906, 29.7769)
  arc A1418 (11.8525, 29.7769) -> (11.9287, 29.7769) centre (11.8906, 29.7769) ccw
  arc A1419 (11.9186, 31.1069) -> (11.8424, 31.1069) centre (11.8805, 31.1069) ccw
  line L709 (11.8874, 22.5601) -> (11.8867, 21.2301)
  arc A1420 (11.8486, 21.2301) -> (11.9248, 21.2301) centre (11.8867, 21.2301) ccw
  arc A1421 (11.9255, 22.5601) -> (11.8493, 22.5601) centre (11.8874, 22.5601) ccw
  line L710 (11.7348, 31.1217) -> (11.7348, 29.8191)
  arc A1422 (11.6967, 29.8191) -> (11.7729, 29.8191) centre (11.7348, 29.8191) ccw
  arc A1423 (11.7729, 31.1217) -> (11.6967, 31.1217) centre (11.7348, 31.1217) ccw
  line L711 (11.7348, 22.5049) -> (11.7348, 21.2023)
  arc A1424 (11.6967, 21.2023) -> (11.7729, 21.2023) centre (11.7348, 21.2023) ccw
  arc A1425 (11.7729, 22.5049) -> (11.6967, 22.5049) centre (11.7348, 22.5049) ccw
  line L712 (11.5757, 31.155) -> (11.5851, 29.8635)
  arc A1426 (11.547, 29.8635) -> (11.6232, 29.8635) centre (11.5851, 29.8635) ccw
  arc A1427 (11.6138, 31.155) -> (11.5376, 31.155) centre (11.5757, 31.155) ccw
  line L713 (11.5825, 22.4713) -> (11.582, 21.1742)
  arc A1428 (11.5439, 21.1742) -> (11.6201, 21.1742) centre (11.582, 21.1742) ccw
  arc A1429 (11.6206, 22.4713) -> (11.5444, 22.4713) centre (11.5825, 22.4713) ccw
  line L714 (11.4226, 31.1876) -> (11.4325, 29.8955)
  arc A1430 (11.3944, 29.8955) -> (11.4706, 29.8955) centre (11.4325, 29.8955) ccw
  arc A1431 (11.4607, 31.1876) -> (11.3845, 31.1876) centre (11.4226, 31.1876) ccw
  line L715 (11.4301, 22.4382) -> (11.4295, 21.1461)
  arc A1432 (11.3914, 21.1461) -> (11.4676, 21.1461) centre (11.4295, 21.1461) ccw
  arc A1433 (11.4682, 22.4382) -> (11.392, 22.4382) centre (11.4301, 22.4382) ccw
  line L716 (11.27, 31.214) -> (11.2798, 29.9275)
  arc A1434 (11.2417, 29.9275) -> (11.3179, 29.9275) centre (11.2798, 29.9275) ccw
  arc A1435 (11.3081, 31.214) -> (11.2319, 31.214) centre (11.27, 31.214) ccw
  line L717 (11.2777, 22.4051) -> (11.2771, 21.1186)
  arc A1436 (11.239, 21.1186) -> (11.3152, 21.1186) centre (11.2771, 21.1186) ccw
  arc A1437 (11.3158, 22.4051) -> (11.2396, 22.4051) centre (11.2777, 22.4051) ccw
  line L718 (11.1215, 31.2251) -> (11.1453, 29.9503)
  arc A1438 (11.1072, 29.9503) -> (11.1834, 29.9503) centre (11.1453, 29.9503) ccw
  arc A1439 (11.1596, 31.2251) -> (11.0834, 31.2251) centre (11.1215, 31.2251) ccw
  line L719 (11.1258, 22.3843) -> (11.1249, 21.1092)
  arc A1440 (11.0868, 21.1092) -> (11.163, 21.1092) centre (11.1249, 21.1092) ccw
  arc A1441 (11.1639, 22.3843) -> (11.0877, 22.3843) centre (11.1258, 22.3843) ccw
  line L720 (10.969, 31.2315) -> (10.9748, 29.9568)
  arc A1442 (10.9367, 29.9568) -> (11.0129, 29.9568) centre (10.9748, 29.9568) ccw
  arc A1443 (11.0071, 31.2315) -> (10.9309, 31.2315) centre (10.969, 31.2315) ccw
  line L721 (10.9729, 22.3736) -> (10.9725, 21.1001)
  arc A1444 (10.9344, 21.1001) -> (11.0106, 21.1001) centre (10.9725, 21.1001) ccw
  arc A1445 (11.011, 22.3736) -> (10.9348, 22.3736) centre (10.9729, 22.3736) ccw
  line L722 (10.8126, 31.238) -> (10.8223, 29.9665)
  arc A1446 (10.7842, 29.9665) -> (10.8604, 29.9665) centre (10.8223, 29.9665) ccw
  arc A1447 (10.8507, 31.238) -> (10.7745, 31.238) centre (10.8126, 31.238) ccw
  line L723 (10.8205, 22.3628) -> (10.8198, 21.091)
  arc A1448 (10.7817, 21.091) -> (10.8579, 21.091) centre (10.8198, 21.091) ccw
  arc A1449 (10.8586, 22.3628) -> (10.7824, 22.3628) centre (10.8205, 22.3628) ccw
  line L724 (10.6676, 31.2441) -> (10.6698, 29.9763)
  arc A1450 (10.6317, 29.9763) -> (10.7079, 29.9763) centre (10.6698, 29.9763) ccw
  arc A1451 (10.7057, 31.2441) -> (10.6295, 31.2441) centre (10.6676, 31.2441) ccw
  line L725 (10.6681, 22.3519) -> (10.668, 21.0819)
  arc A1452 (10.6299, 21.0819) -> (10.7061, 21.0819) centre (10.668, 21.0819) ccw
  arc A1453 (10.7062, 22.3519) -> (10.63, 22.352) centre (10.6681, 22.3519) ccw
  line L726 (10.5152, 31.2364) -> (10.5175, 29.9688)
  arc A1454 (10.4794, 29.9688) -> (10.5556, 29.9688) centre (10.5175, 29.9688) ccw
  arc A1455 (10.5533, 31.2364) -> (10.4771, 31.2364) centre (10.5152, 31.2364) ccw
  line L727 (10.5157, 22.352) -> (10.5156, 21.0955)
  arc A1456 (10.4775, 21.0955) -> (10.5537, 21.0955) centre (10.5156, 21.0955) ccw
  arc A1457 (10.5538, 22.352) -> (10.4776, 22.352) centre (10.5157, 22.352) ccw
  line L728 (10.3629, 31.2287) -> (10.3651, 29.9613)
  arc A1458 (10.327, 29.9613) -> (10.4032, 29.9613) centre (10.3651, 29.9613) ccw
  arc A1459 (10.401, 31.2287) -> (10.3248, 31.2287) centre (10.3629, 31.2287) ccw
  line L729 (10.3633, 22.3574) -> (10.3632, 21.1091)
  arc A1460 (10.3251, 21.1091) -> (10.4013, 21.1091) centre (10.3632, 21.1091) ccw
  arc A1461 (10.4014, 22.3574) -> (10.3252, 22.3574) centre (10.3633, 22.3574) ccw
  line L730 (10.2105, 31.221) -> (10.2142, 29.9538)
  arc A1462 (10.1761, 29.9538) -> (10.2523, 29.9538) centre (10.2142, 29.9538) ccw
  arc A1463 (10.2486, 31.221) -> (10.1724, 31.221) centre (10.2105, 31.221) ccw
  line L731 (10.2108, 22.3736) -> (10.2108, 21.1228)
  arc A1464 (10.1727, 21.1228) -> (10.2489, 21.1228) centre (10.2108, 21.1228) ccw
  arc A1465 (10.2489, 22.3736) -> (10.1727, 22.3736) centre (10.2108, 22.3736) ccw
  line L732 (10.0579, 31.2133) -> (10.059, 29.9307)
  arc A1466 (10.0209, 29.9307) -> (10.0971, 29.9307) centre (10.059, 29.9307) ccw
  arc A1467 (10.096, 31.2133) -> (10.0198, 31.2133) centre (10.0579, 31.2133) ccw
  line L733 (10.0584, 22.3898) -> (10.0584, 21.1364)
  arc A1468 (10.0203, 21.1364) -> (10.0965, 21.1364) centre (10.0584, 21.1364) ccw
  arc A1469 (10.0965, 22.3898) -> (10.0203, 22.3898) centre (10.0584, 22.3898) ccw
  line L734 (9.9059, 31.1913) -> (9.9066, 29.904)
  arc A1470 (9.8685, 29.904) -> (9.9447, 29.904) centre (9.9066, 29.904) ccw
  arc A1471 (9.944, 31.1913) -> (9.8678, 31.1913) centre (9.9059, 31.1913) ccw
  line L735 (9.906, 22.406) -> (9.906, 21.1635)
  arc A1472 (9.8679, 21.1635) -> (9.9441, 21.1635) centre (9.906, 21.1635) ccw
  arc A1473 (9.9441, 22.406) -> (9.8679, 22.406) centre (9.906, 22.406) ccw
  line L736 (9.7535, 31.1637) -> (9.7542, 29.8774)
  arc A1474 (9.7161, 29.8774) -> (9.7923, 29.8774) centre (9.7542, 29.8774) ccw
  arc A1475 (9.7916, 31.1637) -> (9.7154, 31.1637) centre (9.7535, 31.1637) ccw
  line L737 (9.7536, 22.4425) -> (9.7536, 21.1969)
  arc A1476 (9.7155, 21.1969) -> (9.7917, 21.1969) centre (9.7536, 21.1969) ccw
  arc A1477 (9.7917, 22.4425) -> (9.7155, 22.4425) centre (9.7536, 22.4425) ccw
  line L738 (9.6011, 31.1362) -> (9.6012, 29.8367)
  arc A1478 (9.5631, 29.8367) -> (9.6393, 29.8367) centre (9.6012, 29.8367) ccw
  arc A1479 (9.6392, 31.1362) -> (9.563, 31.1362) centre (9.6011, 31.1362) ccw
  line L739 (9.6012, 22.4812) -> (9.6012, 21.2303)
  arc A1480 (9.5631, 21.2303) -> (9.6393, 21.2303) centre (9.6012, 21.2303) ccw
  arc A1481 (9.6393, 22.4812) -> (9.5631, 22.4812) centre (9.6012, 22.4812) ccw
  line L740 (9.4488, 31.1086) -> (9.4488, 29.789)
  arc A1482 (9.4107, 29.789) -> (9.4869, 29.789) centre (9.4488, 29.789) ccw
  arc A1483 (9.4869, 31.1086) -> (9.4107, 31.1086) centre (9.4488, 31.1086) ccw
  line L741 (9.4488, 22.5199) -> (9.4488, 21.2637)
  arc A1484 (9.4107, 21.2637) -> (9.4869, 21.2637) centre (9.4488, 21.2637) ccw
  arc A1485 (9.4869, 22.5199) -> (9.4107, 22.5199) centre (9.4488, 22.5199) ccw
  line L742 (9.2963, 31.0703) -> (9.2964, 29.7413)
  arc A1486 (9.2583, 29.7413) -> (9.3345, 29.7413) centre (9.2964, 29.7413) ccw
  arc A1487 (9.3344, 31.0703) -> (9.2582, 31.0703) centre (9.2963, 31.0703) ccw
  line L743 (9.2935, 22.572) -> (9.2962, 21.3065)
  arc A1488 (9.2581, 21.3065) -> (9.3343, 21.3065) centre (9.2962, 21.3065) ccw
  arc A1489 (9.3316, 22.572) -> (9.2554, 22.572) centre (9.2935, 22.572) ccw
  line L744 (9.144, 31.0217) -> (9.144, 29.6795)
  arc A1490 (9.1059, 29.6795) -> (9.1821, 29.6795) centre (9.144, 29.6795) ccw
  arc A1491 (9.1821, 31.0217) -> (9.1059, 31.0217) centre (9.144, 31.0217) ccw
  line L745 (9.144, 22.635) -> (9.1437, 21.3604)
  arc A1492 (9.1056, 21.3604) -> (9.1818, 21.3604) centre (9.1437, 21.3604) ccw
  arc A1493 (9.1821, 22.635) -> (9.1059, 22.635) centre (9.144, 22.635) ccw
  line L746 (8.9917, 30.973) -> (8.9916, 29.6089)
  arc A1494 (8.9535, 29.6089) -> (9.0297, 29.6089) centre (8.9916, 29.6089) ccw
  arc A1495 (9.0298, 30.973) -> (8.9536, 30.973) centre (8.9917, 30.973) ccw
  line L747 (8.9885, 22.6972) -> (8.9912, 21.4144)
  arc A1496 (8.9531, 21.4144) -> (9.0293, 21.4144) centre (8.9912, 21.4144) ccw
  arc A1497 (9.0266, 22.6972) -> (8.9504, 22.6972) centre (8.9885, 22.6972) ccw
  line L748 (8.8391, 30.9242) -> (8.8392, 29.5382)
  arc A1498 (8.8011, 29.5382) -> (8.8773, 29.5382) centre (8.8392, 29.5382) ccw
  arc A1499 (8.8772, 30.9242) -> (8.801, 30.9242) centre (8.8391, 30.9242) ccw
  line L749 (8.8392, 22.7709) -> (8.8392, 21.4694)
  arc A1500 (8.8011, 21.4694) -> (8.8773, 21.4694) centre (8.8392, 21.4694) ccw
  arc A1501 (8.8773, 22.7709) -> (8.8011, 22.7709) centre (8.8392, 22.7709) ccw
  line L750 (8.6868, 30.8657) -> (8.6868, 29.449)
  arc A1502 (8.6487, 29.449) -> (8.7249, 29.449) centre (8.6868, 29.449) ccw
  arc A1503 (8.7249, 30.8657) -> (8.6487, 30.8657) centre (8.6868, 30.8657) ccw
  line L751 (8.6868, 22.8611) -> (8.6863, 21.5312)
  arc A1504 (8.6482, 21.5312) -> (8.7244, 21.5312) centre (8.6863, 21.5312) ccw
  arc A1505 (8.7249, 22.8611) -> (8.6487, 22.8611) centre (8.6868, 22.8611) ccw
  line L752 (8.5343, 30.7939) -> (8.5344, 29.3523)
  arc A1506 (8.4963, 29.3523) -> (8.5725, 29.3523) centre (8.5344, 29.3523) ccw
  arc A1507 (8.5724, 30.7939) -> (8.4962, 30.7939) centre (8.5343, 30.7939) ccw
  line L753 (8.5344, 22.9512) -> (8.5344, 21.6096)
  arc A1508 (8.4963, 21.6096) -> (8.5725, 21.6096) centre (8.5344, 21.6096) ccw
  arc A1509 (8.5725, 22.9512) -> (8.4963, 22.9512) centre (8.5344, 22.9512) ccw
  line L754 (8.3819, 30.7221) -> (8.382, 29.2552)
  arc A1510 (8.3439, 29.2552) -> (8.4201, 29.2552) centre (8.382, 29.2552) ccw
  arc A1511 (8.42, 30.7221) -> (8.3438, 30.7221) centre (8.3819, 30.7221) ccw
  line L755 (8.382, 23.0543) -> (8.3818, 21.6863)
  arc A1512 (8.3437, 21.6863) -> (8.4199, 21.6863) centre (8.3818, 21.6863) ccw
  arc A1513 (8.4201, 23.0543) -> (8.3439, 23.0543) centre (8.382, 23.0543) ccw
  line L756 (8.2296, 30.6503) -> (8.2296, 29.1279)
  arc A1514 (8.1915, 29.1279) -> (8.2677, 29.1279) centre (8.2296, 29.1279) ccw
  arc A1515 (8.2677, 30.6503) -> (8.1915, 30.6503) centre (8.2296, 30.6503) ccw
  line L757 (8.2296, 23.1768) -> (8.2296, 21.7639)
  arc A1516 (8.1915, 21.7639) -> (8.2677, 21.7639) centre (8.2296, 21.7639) ccw
  arc A1517 (8.2677, 23.1768) -> (8.1915, 23.1768) centre (8.2296, 23.1768) ccw
  line L758 (8.0772, 30.5642) -> (8.0772, 29.0005)
  arc A1518 (8.0391, 29.0005) -> (8.1153, 29.0005) centre (8.0772, 29.0005) ccw
  arc A1519 (8.1153, 30.5642) -> (8.0391, 30.5642) centre (8.0772, 30.5642) ccw
  line L759 (8.0772, 23.2993) -> (8.0773, 21.8546)
  arc A1520 (8.0392, 21.8546) -> (8.1154, 21.8546) centre (8.0773, 21.8546) ccw
  arc A1521 (8.1153, 23.2993) -> (8.0391, 23.2993) centre (8.0772, 23.2993) ccw
  line L760 (7.9248, 30.4662) -> (7.9248, 28.8516)
  arc A1522 (7.8867, 28.8516) -> (7.9629, 28.8516) centre (7.9248, 28.8516) ccw
  arc A1523 (7.9629, 30.4662) -> (7.8867, 30.4662) centre (7.9248, 30.4662) ccw
  line L761 (7.9248, 23.4508) -> (7.9249, 21.9578)
  arc A1524 (7.8868, 21.9578) -> (7.963, 21.9578) centre (7.9249, 21.9578) ccw
  arc A1525 (7.9629, 23.4508) -> (7.8867, 23.4508) centre (7.9248, 23.4508) ccw
  line L762 (7.7724, 30.3683) -> (7.7724, 28.6859)
  arc A1526 (7.7343, 28.6859) -> (7.8105, 28.6859) centre (7.7724, 28.6859) ccw
  arc A1527 (7.8105, 30.3683) -> (7.7343, 30.3683) centre (7.7724, 30.3683) ccw
  line L763 (7.7724, 23.6141) -> (7.7724, 22.061)
  arc A1528 (7.7343, 22.061) -> (7.8105, 22.061) centre (7.7724, 22.061) ccw
  arc A1529 (7.8105, 23.6141) -> (7.7343, 23.6141) centre (7.7724, 23.6141) ccw
  line L764 (7.62, 30.2703) -> (7.62, 28.4999)
  arc A1530 (7.5819, 28.4999) -> (7.6581, 28.4999) centre (7.62, 28.4999) ccw
  arc A1531 (7.6581, 30.2703) -> (7.5819, 30.2703) centre (7.62, 30.2703) ccw
  line L765 (7.62, 23.7973) -> (7.62, 22.1642)
  arc A1532 (7.5819, 22.1642) -> (7.6581, 22.1642) centre (7.62, 22.1642) ccw
  arc A1533 (7.6581, 23.7973) -> (7.5819, 23.7973) centre (7.62, 23.7973) ccw
  line L766 (7.4676, 30.1432) -> (7.4676, 28.2832)
  arc A1534 (7.4295, 28.2832) -> (7.5057, 28.2832) centre (7.4676, 28.2832) ccw
  arc A1535 (7.5057, 30.1432) -> (7.4295, 30.1432) centre (7.4676, 30.1432) ccw
  line L767 (7.4676, 24.0162) -> (7.4676, 22.2963)
  arc A1536 (7.4295, 22.2963) -> (7.5057, 22.2963) centre (7.4676, 22.2963) ccw
  arc A1537 (7.5057, 24.0162) -> (7.4295, 24.0162) centre (7.4676, 24.0162) ccw
  line L768 (7.3152, 30.0143) -> (7.3152, 28.0245)
  arc A1538 (7.2771, 28.0245) -> (7.3533, 28.0245) centre (7.3152, 28.0245) ccw
  arc A1539 (7.3533, 30.0143) -> (7.2771, 30.0143) centre (7.3152, 30.0143) ccw
  line L769 (7.3152, 24.2678) -> (7.3152, 22.4305)
  arc A1540 (7.2771, 22.4305) -> (7.3533, 22.4305) centre (7.3152, 22.4305) ccw
  arc A1541 (7.3533, 24.2678) -> (7.2771, 24.2678) centre (7.3152, 24.2678) ccw
  line L770 (7.1628, 29.8854) -> (7.2084, 27.7423)
  arc A1542 (7.1703, 27.7423) -> (7.2465, 27.7423) centre (7.2084, 27.7423) ccw
  arc A1543 (7.2009, 29.8854) -> (7.1247, 29.8854) centre (7.1628, 29.8854) ccw
  line L771 (7.1628, 24.5713) -> (7.1628, 22.5647)
  arc A1544 (7.1247, 22.5647) -> (7.2009, 22.5647) centre (7.1628, 22.5647) ccw
  arc A1545 (7.2009, 24.5713) -> (7.1247, 24.5713) centre (7.1628, 24.5713) ccw
  line L772 (7.0104, 29.7304) -> (7.6135, 27.563)
  arc A1546 (7.5754, 27.563) -> (7.6516, 27.563) centre (7.6135, 27.563) ccw
  arc A1547 (7.0485, 29.7304) -> (6.9723, 29.7304) centre (7.0104, 29.7304) ccw
  line L773 (7.0104, 25.0026) -> (7.0104, 22.7253)
  arc A1548 (6.9723, 22.7253) -> (7.0485, 22.7253) centre (7.0104, 22.7253) ccw
  arc A1549 (7.0485, 25.0026) -> (6.9723, 25.0026) centre (7.0104, 25.0026) ccw
  line L774 (6.858, 29.5628) -> (6.858, 26.3398)
  arc A1550 (6.8199, 26.3398) -> (6.8961, 26.3398) centre (6.858, 26.3398) ccw
  arc A1551 (6.8961, 29.5628) -> (6.8199, 29.5628) centre (6.858, 29.5628) ccw
  line L775 (6.858, 26.162) -> (6.858, 22.8983)
  arc A1552 (6.8199, 22.8983) -> (6.8961, 22.8983) centre (6.858, 22.8983) ccw
  arc A1553 (6.8961, 26.162) -> (6.8199, 26.162) centre (6.858, 26.162) ccw
  line L776 (6.7056, 29.3951) -> (6.7056, 26.3398)
  arc A1554 (6.6675, 26.3398) -> (6.7437, 26.3398) centre (6.7056, 26.3398) ccw
  arc A1555 (6.7437, 29.3951) -> (6.6675, 29.3951) centre (6.7056, 29.3951) ccw
  line L777 (6.7056, 26.162) -> (6.7056, 23.0713)
  arc A1556 (6.6675, 23.0713) -> (6.7437, 23.0713) centre (6.7056, 23.0713) ccw
  arc A1557 (6.7437, 26.162) -> (6.6675, 26.162) centre (6.7056, 26.162) ccw
  line L778 (6.5532, 29.1865) -> (6.5532, 26.3398)
  arc A1558 (6.5151, 26.3398) -> (6.5913, 26.3398) centre (6.5532, 26.3398) ccw
  arc A1559 (6.5913, 29.1865) -> (6.5151, 29.1865) centre (6.5532, 29.1865) ccw
  line L779 (6.5532, 26.162) -> (6.5532, 23.2868)
  arc A1560 (6.5151, 23.2868) -> (6.5913, 23.2868) centre (6.5532, 23.2868) ccw
  arc A1561 (6.5913, 26.162) -> (6.5151, 26.162) centre (6.5532, 26.162) ccw
  line L780 (6.4008, 28.967) -> (6.4008, 26.3398)
  arc A1562 (6.3627, 26.3398) -> (6.4389, 26.3398) centre (6.4008, 26.3398) ccw
  arc A1563 (6.4389, 28.967) -> (6.3627, 28.967) centre (6.4008, 28.967) ccw
  line L781 (6.4008, 26.162) -> (6.4008, 23.5117)
  arc A1564 (6.3627, 23.5117) -> (6.4389, 23.5117) centre (6.4008, 23.5117) ccw
  arc A1565 (6.4389, 26.162) -> (6.3627, 26.162) centre (6.4008, 26.162) ccw
  line L782 (6.2484, 28.7212) -> (6.2484, 26.3398)
  arc A1566 (6.2103, 26.3398) -> (6.2865, 26.3398) centre (6.2484, 26.3398) ccw
  arc A1567 (6.2865, 28.7212) -> (6.2103, 28.7212) centre (6.2484, 28.7212) ccw
  line L783 (6.2484, 26.162) -> (6.2484, 23.7661)
  arc A1568 (6.2103, 23.7661) -> (6.2865, 23.7661) centre (6.2484, 23.7661) ccw
  arc A1569 (6.2865, 26.162) -> (6.2103, 26.162) centre (6.2484, 26.162) ccw
  line L784 (6.096, 28.4255) -> (6.096, 26.3398)
  arc A1570 (6.0579, 26.3398) -> (6.1341, 26.3398) centre (6.096, 26.3398) ccw
  arc A1571 (6.1341, 28.4255) -> (6.0579, 28.4255) centre (6.096, 28.4255) ccw
  line L785 (6.096, 26.162) -> (6.096, 24.067)
  arc A1572 (6.0579, 24.067) -> (6.1341, 24.067) centre (6.096, 24.067) ccw
  arc A1573 (6.1341, 26.162) -> (6.0579, 26.162) centre (6.096, 26.162) ccw
  line L786 (5.9436, 28.0807) -> (5.9436, 26.3398)
  arc A1574 (5.9055, 26.3398) -> (5.9817, 26.3398) centre (5.9436, 26.3398) ccw
  arc A1575 (5.9817, 28.0807) -> (5.9055, 28.0807) centre (5.9436, 28.0807) ccw
  line L787 (5.9436, 26.162) -> (5.9436, 24.4226)
  arc A1576 (5.9055, 24.4226) -> (5.9817, 24.4226) centre (5.9436, 24.4226) ccw
  arc A1577 (5.9817, 26.162) -> (5.9055, 26.162) centre (5.9436, 26.162) ccw
  line L788 (5.7912, 27.6567) -> (5.7912, 26.3398)
  arc A1578 (5.7531, 26.3398) -> (5.8293, 26.3398) centre (5.7912, 26.3398) ccw
  arc A1579 (5.8293, 27.6567) -> (5.7531, 27.6567) centre (5.7912, 27.6567) ccw
  line L789 (5.7912, 26.162) -> (5.7912, 24.8504)
  arc A1580 (5.7531, 24.8504) -> (5.8293, 24.8504) centre (5.7912, 24.8504) ccw
  arc A1581 (5.8293, 26.162) -> (5.7531, 26.162) centre (5.7912, 26.162) ccw
  line L790 (5.6388, 26.9485) -> (5.6388, 26.3398)
  arc A1582 (5.6007, 26.3398) -> (5.6769, 26.3398) centre (5.6388, 26.3398) ccw
  arc A1583 (5.6769, 26.9485) -> (5.6007, 26.9485) centre (5.6388, 26.9485) ccw
  line L791 (5.6388, 26.162) -> (5.6388, 25.5924)
  arc A1584 (5.6007, 25.5924) -> (5.6769, 25.5924) centre (5.6388, 25.5924) ccw
  arc A1585 (5.6769, 26.162) -> (5.6007, 26.162) centre (5.6388, 26.162) ccw
  line L792 (5.588, 26.3398) -> (5.6423, 26.9905)
  arc A1586 (5.6803, 26.9873) -> (5.6043, 26.9937) centre (5.6423, 26.9905) ccw
  arc A1587 (5.55, 26.343) -> (5.626, 26.3366) centre (5.588, 26.3398) ccw
  line L793 (5.6423, 26.9905) -> (5.7811, 27.6286)
  arc A1588 (5.8183, 27.6205) -> (5.7439, 27.6366) centre (5.7811, 27.6286) ccw
  arc A1589 (5.6051, 26.9986) -> (5.6795, 26.9824) centre (5.6423, 26.9905) ccw
  line L794 (5.7811, 27.6286) -> (6.0019, 28.243)
  arc A1590 (6.0378, 28.2302) -> (5.9661, 28.2559) centre (6.002, 28.243) ccw
  arc A1591 (5.7452, 27.6414) -> (5.8169, 27.6157) centre (5.7811, 27.6286) ccw
  line L795 (6.0019, 28.243) -> (6.3011, 28.8234)
  arc A1592 (6.335, 28.806) -> (6.2673, 28.8409) centre (6.3011, 28.8234) ccw
  arc A1593 (5.9681, 28.2605) -> (6.0358, 28.2256) centre (6.0019, 28.243) ccw
  line L796 (6.3011, 28.8234) -> (6.6735, 29.3598)
  arc A1594 (6.7048, 29.3381) -> (6.6422, 29.3815) centre (6.6735, 29.3598) ccw
  arc A1595 (6.2698, 28.8452) -> (6.3324, 28.8017) centre (6.3011, 28.8234) ccw
  line L797 (6.6735, 29.3598) -> (7.1127, 29.843)
  arc A1596 (7.1409, 29.8174) -> (7.0845, 29.8686) centre (7.1127, 29.843) ccw